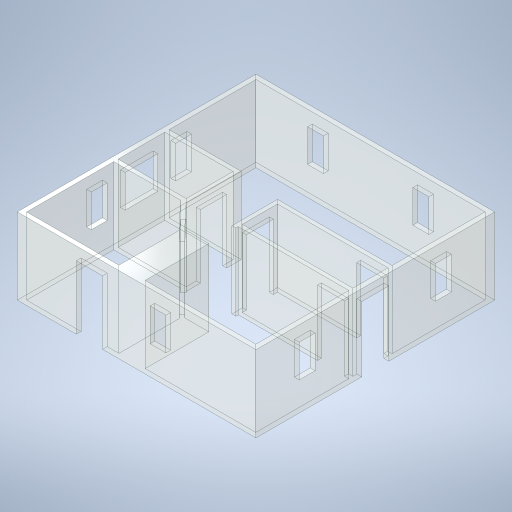
# Autodesk Inventor part: Existing_Kitchen_And_Dining_Room
Saved by Autodesk Inventor 2024 (Build 280153000, 153)
## iProperties
Created: 2023-04-15
Part Number: Existing_Kitchen_And_Dining_Room
Material: Wood (Southern Pine)
Document SubType Name: Modeling
Designer: Tom
Density: 7.85 g/cm^3
Appearance: Clear
Author: Tom
Autodesk Inventor part; units mm, degrees
ref_plane "YZ Plane" through (0, 0, 0) normal (1, 0, 0) x (0, 1, 0)
ref_plane "XZ Plane" through (0, 0, 0) normal (0, 1, 0) x (-1, 0, 0)
ref_plane "XY Plane" through (0, 0, 0) normal (0, 0, 1) x (1, 0, 0)
sketch "Sketch1" plane through (0, 0, 0) normal (0, 1, 0) x (-1, 0, 0)
  line L0 (149.225, -7470.775) -> (149.225, 149.225)
  line L1 (149.225, 149.225) -> (-7470.775, 149.225)
  line L2 (-7470.775, 149.225) -> (-7470.775, -7470.775)
  line L3 (-7470.775, -7470.775) -> (149.225, -7470.775)
  line L4 (149.225, -2419.7869) -> (149.225, -2572.0547)
  line L5 (0, -7321.55) -> (-7315.2, -7321.55)
  line L6 (-7315.2, 0) -> (0, 0)
  line L7 (0, -2781.3) -> (-2133.6, -2781.3)
  line L8 (-2133.6, -2781.3) -> (-2946.4, -1917.7)
  line L9 (-2946.4, -1917.7) -> (-2946.4, 0)
  line L10 (-2178.05, -2914.65) -> (-2178.05, -4413.25)
  line L11 (0, -4546.6) -> (-2305.05, -4546.6)
  line L12 (-2305.05, -4546.6) -> (-2305.05, -2784.4372)
  line L13 (-2305.05, -2784.4372) -> (-3013.2262, -2032)
  line L14 (-3013.2262, -2032) -> (-3784.6, -2032)
  line L15 (-3784.6, -2032) -> (-3784.6, 0)
  line L16 (0, 149.225) -> (0, -7470.775)
  line L17 (0, -2781.3) -> (0, -2684.6127)
  line L18 (0, -4449.9127) -> (0, -4546.6)
  line L19 (0, 149.225) -> (149.225, 149.225)
  line L20 (0, -7470.775) -> (149.225, -7470.775)
  line L21 (-2178.05, -2914.65) -> (0, -2917.825)
  line L22 (-2178.05, -4413.25) -> (0, -4410.075)
  line L23 (0, -2917.825) -> (0, -2781.3)
  line L24 (0, -4410.075) -> (0, -4546.6)
  line L25 (-7315.2, 0) -> (-7315.2, -7321.55)
  line L26 (0, -7321.55) -> (0, -7470.775)
  line L27 (-7315.2, -2971.8) -> (-7315.2, -3098.8)
  line L28 (-7315.2, -4419.6) -> (-7315.2, -4222.75)
  line L29 (-7315.2, -4349.75) -> (-3657.6, -4349.75)
  line L30 (-3657.6, -4349.75) -> (-3657.6, -2895.6)
  line L31 (-3657.6, -2895.6) -> (-3784.6, -2895.6)
  line L32 (-3784.6, -2895.6) -> (-3784.6, -2971.8)
  line L33 (-3784.6, -2971.8) -> (-7315.2, -2971.8)
  line L34 (-7315.2, -3098.8) -> (-3784.6, -3098.8)
  line L35 (-3784.6, -3098.8) -> (-3784.6, -4222.75)
  line L36 (-3784.6, -4222.75) -> (-7315.2, -4222.75)
  line L37 (-7315.2, -4349.75) -> (-7315.2, -4222.75)
  line L38 (-7315.2, -3098.8) -> (-7315.2, -2971.8)
  dimension "d153" = 7620
  dimension "d154" = 149.225
  dimension "d156" = 2774.95
  dimension "d157" = 2781.3
  dimension "d160" = 2305.05
  dimension "d161" = 1492.25
  dimension "d164" = 2178.05
  dimension "d165" = 1498.6
  dimension "d166" = 149.225
  dimension "d167" = 7315.2
  dimension "d168" = 2133.6
  dimension "d169" = 2946.4
  dimension "d170" = 1917.7
  dimension "d175" = 127
  dimension "d180" = 127
  dimension "d181" = 76.2
  dimension "d183" = 2971.8
  dimension "d184" = 2971.8
  dimension "d185" = 3657.6
  dimension "d186" = 2032
  constraints: 76 end point, 12 point on line, 10 perpendicular, 9 collinear, 7 equal length, 7 vertical, 4 horizontal, 3 parallel, 1 coincident, 11 other
  measures "d153" distance of L0.start L0.end
  measures "d154" distance of the line from the sketch origin of L0
  measures "d156" distance between parallel lines of L5 L11
  measures "d157" distance between parallel lines of L6 L7
  measures "d160" distance of L11.start L11.end
  measures "d161" distance of L22.end L21.end
  measures "d164" distance of the line from the sketch origin of L10
  measures "d165" distance of L10.start L10.end
  measures "d166" distance between parallel lines of L1 L6
  measures "d167" distance of L5.start L5.end
  measures "d168" distance of L7.start L7.end
  measures "d169" distance of the line from the sketch origin of L9
  measures "d170" distance of L8.end L9.end
  measures "d175" distance between parallel lines of L13 L8
  measures "d180" distance between parallel lines of L33 L34
  measures "d181" distance between parallel lines of L31 L33
  measures "d183" distance between parallel lines of L6 L33
  measures "d184" distance between parallel lines of L5 L29
  measures "d185" distance of L29.start L29.end
  measures "d186" distance of L14.end L15.end
extrude "Extrusion1" add sketch "Sketch1" along normal blind 2438.4 contours L3 L16 L1 L0 | L3 L2 L1 L16 L6 L25 L5 | L11 L12 L13 L14 L15 L6 L9 L8 L7 L16 L21 L10 L22 | L25 L36 L35 L34 L33 L32 L31 L30 L29
sketch "Sketch3" plane through (7470.775, 0, -7470.775) normal (0, 0, -1) x (-1, 0, 0)
  line L0 (5314.95, 1955.8) -> (5822.95, 1955.8)
  line L1 (5822.95, 1955.8) -> (5822.95, 914.4)
  line L2 (5822.95, 914.4) -> (5314.95, 914.4)
  line L3 (5314.95, 914.4) -> (5314.95, 1955.8)
  line L4 (0, 0) -> (7620, 0) projected
  line L5 (1952.625, 1955.8) -> (2460.625, 1955.8)
  line L6 (2460.625, 1955.8) -> (2460.625, 914.4)
  line L7 (2460.625, 914.4) -> (1952.625, 914.4)
  line L8 (1952.625, 914.4) -> (1952.625, 1955.8)
  line L9 (155.575, 0) -> (155.575, 2438.4) projected
  line L10 (7620, 0) -> (7620, 2438.4) projected
  dimension "d78" = 1041.4
  dimension "d79" = 508
  dimension "d81" = 2305.05
  dimension "d82" = 1041.4
  dimension "d83" = 508
  dimension "d84" = 914.4
  dimension "d85" = 914.4
  dimension "d234" = 2305.05
  constraints: 16 end point, 4 parallel, 2 horizontal, 2 perpendicular
  measures "d78" distance of L0.end L1.end
  measures "d79" distance of L0.start L0.end
  measures "d81" distance between parallel lines of L9 L6
  measures "d82" distance of L5.end L6.end
  measures "d83" distance of L5.start L5.end
  measures "d84" distance between parallel lines of L4 L7
  measures "d85" distance between parallel lines of L4 L2
  measures "d234" distance between parallel lines of L10 L3
extrude "Extrusion3" cut sketch "Sketch3" against normal up to surface (149.225 mm away)
sketch "Sketch5" plane through (-149.225, 0, 149.225) normal (0, 0, 1) x (1, 0, 0)
  line L0 (0, 0) -> (7620, 0) projected
  line L1 (2724.15, 0) -> (1885.95, 0)
  line L2 (1885.95, 0) -> (1885.95, 2032)
  line L3 (1885.95, 2032) -> (2724.15, 2032)
  line L4 (2724.15, 2032) -> (2724.15, 0)
  line L5 (0, 0) -> (0, 2438.4) projected
  line L6 (4238.625, 1955.8) -> (4746.625, 1955.8)
  line L7 (4746.625, 1955.8) -> (4746.625, 914.4)
  line L8 (4746.625, 914.4) -> (4238.625, 914.4)
  line L9 (4238.625, 914.4) -> (4238.625, 1955.8)
  point P0 (149.225, 0)
  point P1 (3933.825, 2438.4)
  point P2 (1885.95, 0)
  point P3 (149.225, 2438.4)
  dimension "d102" = 838.2
  dimension "d103" = 2032
  dimension "d104" = 304.8
  dimension "d105" = 508
  dimension "d106" = 914.4
  dimension "d107" = 1041.4
  dimension "d114" = 1736.725
  constraints: 16 end point, 4 parallel, 2 horizontal, 2 perpendicular, 1 point on line
  measures "d102" distance between parallel lines of L4 L2
  measures "d103" distance between parallel lines of L0 L3
  measures "d104" distance from line of point (3933.825, 2438.4) L9
  measures "d105" distance of L6.start L6.end
  measures "d106" distance between parallel lines of L0 L8
  measures "d107" distance of L6.end L7.end
  measures "d114" distance from line of L2 point (149.225, 2438.4)
extrude "Extrusion5" cut sketch "Sketch5" against normal up to surface (149.225 mm away)
sketch "Sketch6" plane through (2946.4, 0, -1917.7) normal (-0.7282, 0, 0.6853647) x (0.6853647, 0, 0.7282)
  line L0 (-37.433, 0) -> (-1070.7167, 0) projected
  line L1 (-161.1749, 0) -> (-1024.7749, 0)
  line L2 (-1024.7749, 0) -> (-1024.7749, 2032)
  line L3 (-1024.7749, 2032) -> (-161.1749, 2032)
  line L4 (-161.1749, 2032) -> (-161.1749, 0)
  line L5 (-1185.9379, 0) -> (-1185.9379, 2438.4) projected
  point P0 (-622.8894, 0)
  point P1 (-1024.7749, 0)
  point P2 (-1024.7749, 0)
  dimension "d115" = 863.6
  dimension "d117" = 2032
  dimension "d235" = 161.163
  constraints: 8 end point, 2 parallel, 1 horizontal, 1 perpendicular, 1 point on line
  measures "d115" distance of L2.end L3.end
  measures "d117" distance of L3.end L1.start
  measures "d235" distance between parallel lines of L5 L2
extrude "Extrusion6" cut sketch "Sketch6" against normal up to surface (127 mm away)
sketch "Sketch7" plane through (2305.05, 0, -2784.4372) normal (1, 0, 0) x (0, 0, -1)
  line L0 (1295.2791, 0) -> (457.0791, 0)
  line L1 (457.0791, 0) -> (457.0791, 2032)
  line L2 (457.0791, 2032) -> (1295.2791, 2032)
  line L3 (1295.2791, 2032) -> (1295.2791, 0)
  line L4 (0, 0) -> (1762.1628, 0) projected
  line L5 (1762.1628, 0) -> (1762.1628, 2438.4) projected
  point P0 (-2784.4372, 0)
  dimension "d120" = 838.2
  dimension "d121" = 466.8838
  dimension "d122" = 2032
  constraints: 8 end point, 2 parallel, 1 collinear, 1 horizontal, 1 perpendicular
  measures "d120" distance of L1.end L2.end
  measures "d121" distance between parallel lines of L5 L3
  measures "d122" distance of L2.end L0.start
extrude "Extrusion7" cut sketch "Sketch7" against normal up to surface (127 mm away)
sketch "Sketch11" plane through (-149.225, 0, -7470.775) normal (-1, 0, 0) x (0, 0, 1)
  line L0 (3286.125, 1955.8) -> (4327.525, 1955.8)
  line L1 (4327.525, 1955.8) -> (4327.525, 914.4)
  line L2 (4327.525, 914.4) -> (3286.125, 914.4)
  line L3 (3286.125, 914.4) -> (3286.125, 1955.8)
  line L4 (0, 0) -> (7620, 0) projected
  line L5 (4552.95, 0) -> (4552.95, 2438.4) projected
  point P0 (7470.775, 0)
  dimension "d187" = 914.4
  dimension "d189" = 1041.4
  dimension "d190" = 1041.4
  dimension "d191" = 225.425
  constraints: 8 end point, 2 parallel, 1 horizontal, 1 perpendicular
  measures "d187" distance between parallel lines of L4 L2
  measures "d189" distance of L2.end L0.start
  measures "d190" distance of L0.start L0.end
  measures "d191" distance between parallel lines of L5 L1
extrude "Extrusion11" cut sketch "Sketch11" against normal up to surface (149.225 mm away)
sketch "Sketch12" plane through (-149.225, 0, -7470.775) normal (-1, 0, 0) x (0, 0, 1)
  line L0 (4899.025, 914.4) -> (5407.025, 914.4)
  line L1 (5407.025, 914.4) -> (5407.025, 1955.8)
  line L2 (5407.025, 1955.8) -> (4899.025, 1955.8)
  line L3 (4899.025, 1955.8) -> (4899.025, 914.4)
  line L4 (4689.475, 0) -> (4689.475, 2438.4) projected
  line L5 (0, 0) -> (7620, 0) projected
  line L6 (2714.625, 1955.8) -> (2206.625, 1955.8)
  line L7 (2206.625, 1955.8) -> (2206.625, 914.4)
  line L8 (2206.625, 914.4) -> (2714.625, 914.4)
  line L9 (2714.625, 914.4) -> (2714.625, 1955.8)
  line L10 (2924.175, 0) -> (2924.175, 2438.4) projected
  point P0 (7470.775, 0)
  dimension "d194" = 209.55
  dimension "d195" = 1041.4
  dimension "d196" = 914.4
  dimension "d197" = 508
  dimension "d198" = 209.55
  dimension "d199" = 508
  dimension "d200" = 1041.4
  dimension "d201" = 914.4
  constraints: 16 end point, 4 parallel, 2 horizontal, 2 perpendicular
  measures "d194" distance between parallel lines of L4 L3
  measures "d195" distance of L0.end L1.end
  measures "d196" distance between parallel lines of L5 L0
  measures "d197" distance of L1.end L2.end
  measures "d198" distance between parallel lines of L10 L9
  measures "d199" distance of L6.start L6.end
  measures "d200" distance of L6.end L7.end
  measures "d201" distance between parallel lines of L5 L8
extrude "Extrusion12" cut sketch "Sketch12" against normal up to surface (149.225 mm away)
sketch "Sketch13" plane through (7470.775, 0, 149.225) normal (1, 0, 0) x (0, 0, -1)
  line L0 (4371.975, 0) -> (3248.025, 0) projected
  line L1 (4241.8, 0) -> (3378.2, 0)
  line L2 (3378.2, 0) -> (3378.2, 2082.8)
  line L3 (3378.2, 2082.8) -> (4241.8, 2082.8)
  line L4 (4241.8, 2082.8) -> (4241.8, 0)
  point P0 (149.225, 0)
  point P1 (4371.975, 2438.4)
  dimension "d204" = 863.6
  dimension "d205" = 130.175
  dimension "d206" = 2082.8
  constraints: 8 end point, 2 parallel, 1 horizontal, 1 perpendicular, 1 point on line
  measures "d204" distance of L2.end L3.end
  measures "d205" distance from line of point (4371.975, 2438.4) L4
  measures "d206" distance of L1.end L2.end
extrude "Extrusion13" cut sketch "Sketch13" against normal up to surface (155.575 mm away)
sketch "Sketch14" plane through (7470.775, 0, -7470.775) normal (1, 0, 0) x (0, 0, -1)
  line L0 (-5730.875, 1955.8) -> (-6238.875, 1955.8)
  line L1 (-6238.875, 1955.8) -> (-6238.875, 914.4)
  line L2 (-6238.875, 914.4) -> (-5730.875, 914.4)
  line L3 (-5730.875, 914.4) -> (-5730.875, 1955.8)
  line L4 (-1381.125, 1955.8) -> (-1381.125, 914.4)
  line L5 (-1889.125, 914.4) -> (-1889.125, 1955.8)
  line L6 (-7620, 0) -> (-4241.8, 0) projected
  line L7 (-1889.125, 914.4) -> (-1381.125, 914.4)
  line L8 (-1889.125, 1955.8) -> (-1381.125, 1955.8)
  line L9 (-3378.2, 0) -> (0, 0) projected
  point P0 (-7470.775, 0)
  point P1 (-4498.975, 2438.4)
  point P2 (-5984.875, 914.4)
  point P3 (-3121.025, 2438.4)
  dimension "d210" = 508
  dimension "d212" = 1041.4
  dimension "d214" = 1231.9
  dimension "d216" = 914.4
  dimension "d218" = 1041.4
  dimension "d219" = 508
  dimension "d220" = 1231.9
  dimension "d221" = 914.4
  constraints: 16 end point, 3 horizontal, 3 parallel, 2 perpendicular, 1 midpoint
  measures "d210" distance of L0.start L0.end
  measures "d212" distance of L0.end L1.end
  measures "d214" distance from line of point (-3121.025, 2438.4) L5
  measures "d216" distance between parallel lines of L9 L7
  measures "d218" distance of L4.start L4.end
  measures "d219" distance of L5.end L4.start
  measures "d220" distance from line of point (-4498.975, 2438.4) L3
  measures "d221" distance between parallel lines of L6 L2
extrude "Extrusion14" cut sketch "Sketch14" against normal up to surface (155.575 mm away)
sketch "Sketch15" plane through (3784.6, 0, -3098.8) normal (1, 0, 0) x (0, 0, -1)
  line L0 (1250.95, 0) -> (-203.2, 0) projected
  line L1 (130.175, 0) -> (993.775, 0)
  line L2 (993.775, 0) -> (993.775, 2082.8)
  line L3 (993.775, 2082.8) -> (130.175, 2082.8)
  line L4 (130.175, 2082.8) -> (130.175, 0)
  point P0 (-3098.8, 0)
  point P1 (0, 2438.4)
  point P2 (993.775, 0)
  dimension "d224" = 130.175
  dimension "d225" = 863.6
  dimension "d226" = 2082.8
  constraints: 8 end point, 2 parallel, 1 horizontal, 1 perpendicular, 1 point on line
  measures "d224" distance from line of L4 point (0, 2438.4)
  measures "d225" distance of L2.end L3.end
  measures "d226" distance of L1.end L2.end
extrude "Extrusion15" cut sketch "Sketch15" against normal up to surface (127 mm away)
sketch "Sketch16" plane through (7315.2, 0, -4349.75) normal (0, 0, -1) x (-1, 0, 0)
  line L0 (0, 0) -> (3657.6, 0) projected
  line L1 (139.7, 0) -> (1003.3, 0)
  line L2 (1003.3, 0) -> (1003.3, 2082.8)
  line L3 (1003.3, 2082.8) -> (139.7, 2082.8)
  line L4 (139.7, 2082.8) -> (139.7, 0)
  point P0 (7315.2, 0)
  point P1 (0, 2438.4)
  dimension "d229" = 139.7
  dimension "d230" = 863.6
  dimension "d231" = 2082.8
  constraints: 8 end point, 2 parallel, 1 horizontal, 1 perpendicular, 1 point on line
  measures "d229" distance from line of point (0, 2438.4) L4
  measures "d230" distance of L2.end L3.end
  measures "d231" distance of L1.end L2.end
extrude "Extrusion16" cut sketch "Sketch16" against normal up to surface (1377.95 mm away)
body "Solid1"
